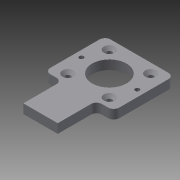
# Autodesk Inventor part: pitch_mount
Saved by Autodesk Inventor 2015 (Build 190159000, 159)
## iProperties
Created: 2015-12-01
Part Number: pitch_mount
Material: Generic
Document SubType Name: Modeling
Designer: jufranz
Density: 1 g/cm^3
Appearance: Default
Author: jufranz
Autodesk Inventor part; units mm, degrees
ref_plane "YZ Plane" through (0, 0, 0) normal (1, 0, 0) x (0, 1, 0)
ref_plane "XZ Plane" through (0, 0, 0) normal (0, 1, 0) x (-1, 0, 0)
ref_plane "XY Plane" through (0, 0, 0) normal (0, 0, 1) x (1, 0, 0)
sketch "Sketch1" plane through (0, 0, 0) normal (0, 1, 0) x (-1, 0, 0)
  line L0 (20, 14.325) -> (20, -14.325)
  line L1 (16.825, -17.5) -> (-16.825, -17.5)
  line L2 (-20, -14.325) -> (-20, 14.325)
  line L3 (-16.825, 17.5) -> (-13.175, 17.5)
  line L4 (-10, 20.675) -> (-10, 40)
  line L5 (-10, 40) -> (10, 40)
  line L6 (10, 40) -> (10, 20.675)
  line L7 (13.175, 17.5) -> (16.825, 17.5)
  arc A0 (10, 20.675) -> (13.175, 17.5) centre (13.175, 20.675) ccw
  arc A1 (-13.175, 17.5) -> (-10, 20.675) centre (-13.175, 20.675) ccw
  arc A2 (20, 14.325) -> (16.825, 17.5) centre (16.825, 14.325) ccw
  arc A3 (16.825, -17.5) -> (20, -14.325) centre (16.825, -14.325) ccw
  arc A4 (-20, -14.325) -> (-16.825, -17.5) centre (-16.825, -14.325) ccw
  arc A5 (-16.825, 17.5) -> (-20, 14.325) centre (-16.825, 14.325) ccw
  point P0 (0, 0)
  point P1 (20, 17.5)
  point P2 (20, -17.5)
  point P3 (-20, -17.5)
  point P4 (-20, 17.5)
  point P5 (-10, 17.5)
  point P6 (10, 17.5)
  point P7 (20, 0)
  point P8 (0, -17.5)
  point P9 (0, 40)
  dimension "d0" = 35
  dimension "d1" = 40
  dimension "d2" = 20
  dimension "d3" = 40
  dimension "d26" = 3.175
  dimension "d27" = 3.175
  constraints: 16 end point, 13 point on line, 12 point on circle, 12 tangent, 7 perpendicular, 6 centre point, 4 equal radius, 3 midpoint, 2 vertical alignment, 1 horizontal alignment, 1 vertical
  measures "d0" distance of point (20, 17.5) point (20, -17.5)
  measures "d1" distance of point (20, -17.5) point (-20, -17.5)
  measures "d2" distance between parallel lines of L4 L6
  measures "d3" distance from line of point (0, 0) L5
  measures "d26" radius of A0
  measures "d27" radius of A2
extrude "Extrusion1" add sketch "Sketch1" along normal blind 5.334
sketch "Sketch2" plane through (0, 5.334, 0) normal (0, 1, 0) x (1, 0, 0)
  line L0 (-12.0208, -12.0208) -> (0, 0)
  line L1 (0, 0) -> (-20, 0)
  line L2 (-20, 14.325) -> (-20, -14.325) projected
  point P0 (-17.5, 17.5)
  point P1 (-17.5, -17.5)
  point P2 (12.0208, -12.0208)
  point P3 (12.0208, 12.0208)
  point P4 (-12.0208, 12.0208)
  dimension "d6" = 17
  dimension "d7" = 45
  dimension "d10" = 360
  constraints: 4 end point, 1 coincident, 7 other
  measures "d6" distance of point (0, 0) L0.start
  measures "d7" angle of L0 L1
hole "Hole1" at (-12.0208, 5.334, 12.0208) at (12.0208, 5.334, 12.0208) at (12.0208, 5.334, -12.0208) at (-12.0208, 5.334, -12.0208) direction (0, -1, 0) diameter 3.2 end through all countersink diameter 6.35 countersink angle 82
sketch "Sketch3" plane through (0, 5.334, 0) normal (0, 1, 0) x (1, 0, 0)
  point P0 (0, 0)
  point P1 (0, 0)
  constraints: 1 coincident
hole "Hole2" at (0, 5.334, 0) direction (0, -1, 0) diameter 20 end through all
sketch "Sketch4" plane through (0, 5.334, 0) normal (0, 1, 0) x (1, 0, 0)
  point P0 (0, 0)
  point P1 (-16.215, 0)
  point P2 (16.215, 0)
  dimension "d28" = 32.43
  dimension "d29" = 16.215
  measures "d28" distance of point (16.215, 0) point (-16.215, 0)
  measures "d29" distance of point (-16.215, 0) point (0, 0)
hole "Hole3" at (-16.215, 5.334, 0) at (16.215, 5.334, 0) direction (0, -1, 0) diameter 2.4638 end through all
equation "\"d29\" = 0.5 * d28"
body "Solid1"
